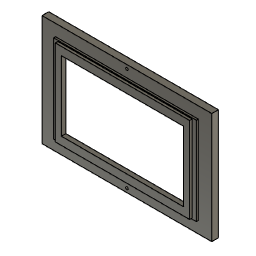
Upper Body (Autodesk Fusion 360 design; units mm, degrees)
Autodesk Fusion 360 part; units mm, degrees
sketch "Sketch1" plane through (0, 0, 0) normal (0, 1, 0) x (1, 0, 0)
  line L0 (55.8, -34.3) -> (-55.8, -34.3)
  line L1 (-55.8, -34.3) -> (-55.8, 34.3)
  line L2 (-55.8, 34.3) -> (55.8, 34.3)
  line L3 (55.8, 34.3) -> (55.8, -34.3)
  line L4 (55.8, -34.3) -> (-55.8, 34.3) construction
  line L5 (-55.8, -34.3) -> (55.8, 34.3) construction
  line L6 (-66.3, -43.35) -> (66.3, -43.35)
  line L7 (66.3, -43.35) -> (66.3, 43.35)
  line L8 (66.3, 43.35) -> (-66.3, 43.35)
  line L9 (-66.3, 43.35) -> (-66.3, -43.35)
  line L10 (-66.3, -43.35) -> (66.3, 43.35) construction
  line L11 (66.3, -43.35) -> (-66.3, 43.35) construction
  circle A0 centre (0, -40.35) radius 1
  circle A1 centre (0, 40.35) radius 1
  point P0 (0, 40.35)
  dimension "d1" = 111.6
  dimension "d2" = 68.6
  dimension "d3" = 132.6
  dimension "d4" = 86.7
  dimension "d12" = 2
  dimension "d13" = 2
  constraint horizontal L0
  constraint perpendicular L0 L1
  constraint parallel L0 L2
  constraint parallel L1 L3
  constraint coincident L4 origin
  constraint coincident L5 origin
  constraint horizontal L6
  constraint perpendicular L6 L7
  constraint parallel L6 L8
  constraint parallel L7 L9
  constraint coincident L10 origin
  constraint coincident L11 origin
  constraint coincident P0 A1.centre
  measures "d1" distance of L1.end L2.end
  measures "d2" distance of L0.end L1.end
  measures "d3" distance of L7.end L8.end
  measures "d4" distance of L6.end L7.end
  measures "d12" diameter of A0
  measures "d13" diameter of A1
extrude "Extrude1" add sketch "Sketch1" along normal blind 5.2 contours L6 L7 L8 L9 | A0 | A1
extrude "Extrude3" cut sketch "Sketch1" along normal blind 20 contours A0 | A1
sketch "Sketch2" plane through (0, 0, 0) normal (0, -1, 0) x (1, 0, 0)
  circle A0 centre (0, -40.35) radius 1
  circle A1 centre (0, 40.35) radius 1
  line L0 (55.8, -34.3) -> (-55.8, -34.3)
  line L1 (-55.8, -34.3) -> (-55.8, 34.3)
  line L2 (-55.8, 34.3) -> (55.8, 34.3)
  line L3 (55.8, 34.3) -> (55.8, -34.3)
  line L4 (-66.3, 43.35) -> (-66.3, -43.35)
  line L5 (-66.3, -43.35) -> (66.3, -43.35)
  line L6 (66.3, -43.35) -> (66.3, 43.35)
  line L7 (66.3, 43.35) -> (-66.3, 43.35)
  line L8 (-47.7, 27.25) -> (47.7, 27.25)
  line L9 (47.7, 27.25) -> (47.7, -27.25)
  line L10 (47.7, -27.25) -> (-47.7, -27.25)
  line L11 (-47.7, -27.25) -> (-47.7, 27.25)
  line L12 (-47.7, 27.25) -> (47.7, -27.25) construction
  line L13 (47.7, 27.25) -> (-47.7, -27.25) construction
  dimension "d16" = 95.4
  dimension "d17" = 54.5
  constraint horizontal L8
  constraint perpendicular L8 L9
  constraint parallel L8 L10
  constraint parallel L9 L11
  constraint coincident L12 origin
  constraint coincident L13 origin
  measures "d16" distance of L9.end L10.end
  measures "d17" distance of L8.end L9.end
extrude "Extrude4" add sketch "Sketch2" along normal blind 3 contours L0 L1 L2 L3
sketch "Sketch3" plane through (0, 0, 0) normal (0, 1, 0) x (1, 0, 0)
sketch "Sketch4" plane through (0, -3, 0) normal (0, -1, 0) x (1, 0, 0)
  line L0 (47.7, -27.25) -> (-47.7, -27.25)
  line L1 (-47.7, -27.25) -> (-47.7, 27.25)
  line L2 (-47.7, 27.25) -> (47.7, 27.25)
  line L3 (47.7, 27.25) -> (47.7, -27.25)
  line L4 (55.8, 34.3) -> (-55.8, 34.3)
  line L5 (-55.8, 34.3) -> (-55.8, -34.3)
  line L6 (-55.8, -34.3) -> (55.8, -34.3)
  line L7 (55.8, -34.3) -> (55.8, 34.3)
  line L8 (-52.5, 33.5) -> (52.5, 33.5)
  line L9 (52.5, 33.5) -> (52.5, -33.5)
  line L10 (52.5, -33.5) -> (-52.5, -33.5)
  line L11 (-52.5, -33.5) -> (-52.5, 33.5)
  line L12 (-52.5, 33.5) -> (52.5, -33.5) construction
  line L13 (52.5, 33.5) -> (-52.5, -33.5) construction
  dimension "d20" = 105
  dimension "d21" = 67
  constraint horizontal L8
  constraint perpendicular L8 L9
  constraint parallel L8 L10
  constraint parallel L9 L11
  constraint coincident L12 origin
  constraint coincident L13 origin
  measures "d20" distance of L9.end L10.end
  measures "d21" distance of L8.end L9.end
extrude "Extrude5" cut 1 faces at (53.1, -3, -9.0833) along direction (0, 1, 0) blind 1.5
sketch "Sketch5" plane through (0, -1.5, 0) normal (0, -1, 0) x (1, 0, 0)
  line L0 (47.7, -27.25) -> (-47.7, -27.25)
  line L1 (-47.7, -27.25) -> (-47.7, 27.25)
  line L2 (-47.7, 27.25) -> (47.7, 27.25)
  line L3 (47.7, 27.25) -> (47.7, -27.25)
  line L4 (55.8, 34.3) -> (-55.8, 34.3)
  line L5 (-55.8, 34.3) -> (-55.8, -34.3)
  line L6 (-55.8, -34.3) -> (55.8, -34.3)
  line L7 (55.8, -34.3) -> (55.8, 34.3)
  line L8 (52.5, 33.5) -> (-52.5, 33.5)
  line L9 (-52.5, 33.5) -> (-52.5, -33.5)
  line L10 (-52.5, -33.5) -> (52.5, -33.5)
  line L11 (52.5, -33.5) -> (52.5, 33.5)
  line L12 (52.5, 33.5) -> (-52.5, -33.5) construction
  line L13 (-52.5, 33.5) -> (52.5, -33.5) construction
  dimension "d24" = 105
  dimension "d25" = 67
  constraint horizontal L8
  constraint perpendicular L8 L9
  constraint parallel L8 L10
  constraint parallel L9 L11
  constraint coincident L12 origin
  constraint coincident L13 origin
  measures "d24" distance of L9.end L10.end
  measures "d25" distance of L8.end L9.end
extrude "Extrude6" add sketch "Sketch4" against normal blind 2 contours L8 L9 L10 L11
extrude "Extrude8" add 1 faces at (15.9, -3, -31.4167) along direction (0, -1, 0) blind 0.5
